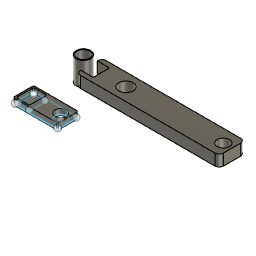
Chocolate Printer Parts v6 (Autodesk Fusion 360 design; units mm, degrees)
Autodesk Fusion 360 part; units mm, degrees
note: some values were not read from the file. Set by a fixed rule: which sketch regions a step uses.
sketch "Sketch1" plane through (0, 0, 0) normal (0, 0, 1) x (1, 0, 0)
  circle A0 centre (0, 0) radius 2.5
  circle A1 centre (0, 0) radius 3
  circle A2 centre (0, 0) radius 6
  circle A3 centre (0, 0) radius 7
  dimension "d1" = 5
  dimension "d2" = 0.5
  dimension "d5" = 12
  dimension "d6" = 1
  constraint coincident A0.centre A1.centre
  constraint concentric A0 A2
  measures "d1" diameter of A0
  measures "d5" diameter of A2
extrude "Extrude1" add sketch "Sketch1" along normal blind 10 contours A3 makes body 1
extrude "Extrude2" add sketch "Sketch1" against normal blind 5 contours A2 | A3 bodies 1
sketch "Sketch2" plane through (0, 0, 0) normal (0, 0, 1) x (1, 0, 0)
  line L0 (17, 5) -> (148.5, 5)
  line L1 (152.5, 1) -> (152.5, -16)
  line L2 (148.5, -20) -> (17, -20)
  line L3 (13, -16) -> (13, 1)
  line L4 (13, 0.5) -> (24, 0.5)
  line L5 (25, -0.5) -> (25, -14.5)
  line L6 (24, -15.5) -> (13, -15.5)
  line L7 (13, -15.5) -> (13, 0.5)
  circle A0 centre (49, -7.5) radius 6.5
  circle A1 centre (49, -7.5) radius 7
  circle A2 centre (144, -7.5) radius 6
  arc A3 (17, 5) -> (13, 1) centre (17, 1) ccw
  arc A4 (13, -16) -> (17, -20) centre (17, -16) ccw
  arc A5 (148.5, -20) -> (152.5, -16) centre (148.5, -16) ccw
  arc A6 (152.5, 1) -> (148.5, 5) centre (148.5, 1) ccw
  arc A7 (25, -0.5) -> (24, 0.5) centre (24, -0.5) ccw
  arc A8 (24, -15.5) -> (25, -14.5) centre (24, -14.5) ccw
  point P0 (12.5, -1.5)
  dimension "d9" = 25
  dimension "d10" = 16
  dimension "d11" = 4.5
  dimension "d12" = 4.5
  dimension "d13" = 12
  dimension "d14" = 24
  dimension "d15" = 13
  dimension "d16" = 0.5
  dimension "d17" = 95
  dimension "d18" = 12.5
  dimension "d19" = 12.5
  dimension "d20" = 12.5
  dimension "d21" = 12.5
  dimension "d22" = 12
  dimension "d39" = 4
  dimension "d40" = 4
  dimension "d41" = 1
  dimension "d47" = 8.5
  constraint horizontal L0
  constraint vertical L1
  constraint horizontal L2
  constraint vertical L3
  constraint horizontal L4
  constraint vertical L5
  constraint horizontal L6
  constraint vertical L7
  constraint coincident L3 L4.start
  constraint tangent L0 A3
  constraint tangent L3 A3
  constraint tangent L2 A4
  constraint tangent L3 A4
  constraint tangent L1 A5
  constraint tangent L2 A5
  constraint equal A4 A5
  constraint tangent L0 A6
  constraint tangent L1 A6
  constraint equal A4 A6
  constraint tangent L4 A7
  constraint tangent L5 A7
  constraint tangent L5 A8
  constraint tangent L6 A8
  constraint equal A7 A8
  measures "d9" distance of L0 L2
  measures "d10" distance of L4 L6
  measures "d11" distance of L0 L4
  measures "d12" distance of L2 L6
  measures "d13" distance of L3 L5
  measures "d14" distance of L5 A0.centre
  measures "d15" diameter of A0
  measures "d17" distance of A0.centre A2.centre
  measures "d18" distance of L0 A0.centre
  measures "d19" distance of L2 A0.centre
  measures "d20" distance of L2 A2.centre
  measures "d21" distance of L0 A2.centre
  measures "d22" diameter of A2
  measures "d39" radius of A3
  measures "d40" radius of A4
  measures "d41" radius of A7
  measures "d47" distance of L1 A2.centre
extrude "Extrude3" add sketch "Sketch2" along normal blind 11 separate body contours L0 L1 L2 L3 L4 L5 L6 A3 A4 A5 A6 A7 A8 makes body 2
sketch "Sketch3" plane through (0, 0, 0) normal (0, 0, 1) x (1, 0, 0)
  line L0 (-2.1132, -45.5462) -> (39.3868, -45.5462)
  line L1 (40.3868, -46.5462) -> (40.3868, -64.5462)
  line L2 (39.3868, -65.5462) -> (-2.1132, -65.5462)
  line L3 (-3.1132, -64.5462) -> (-3.1132, -46.5462)
  line L4 (-0.6132, -47.0462) -> (10.3868, -47.0462)
  line L5 (11.3868, -48.0462) -> (11.3868, -63.0462)
  line L6 (10.3868, -64.0462) -> (-0.6132, -64.0462)
  line L7 (-1.6132, -63.0462) -> (-1.6132, -48.0462)
  circle A0 centre (33.3868, -55.5462) radius 5.5
  arc A1 (-0.6132, -47.0462) -> (-1.6132, -48.0462) centre (-0.6132, -48.0462) ccw
  arc A2 (11.3868, -48.0462) -> (10.3868, -47.0462) centre (10.3868, -48.0462) ccw
  arc A3 (10.3868, -64.0462) -> (11.3868, -63.0462) centre (10.3868, -63.0462) ccw
  arc A4 (-1.6132, -63.0462) -> (-0.6132, -64.0462) centre (-0.6132, -63.0462) ccw
  arc A5 (-2.1132, -45.5462) -> (-3.1132, -46.5462) centre (-2.1132, -46.5462) ccw
  arc A6 (-3.1132, -64.5462) -> (-2.1132, -65.5462) centre (-2.1132, -64.5462) ccw
  arc A7 (39.3868, -65.5462) -> (40.3868, -64.5462) centre (39.3868, -64.5462) ccw
  arc A8 (40.3868, -46.5462) -> (39.3868, -45.5462) centre (39.3868, -46.5462) ccw
  dimension "d25" = 20
  dimension "d26" = 17
  dimension "d27" = 1.5
  dimension "d28" = 1.5
  dimension "d29" = 1.5
  dimension "d30" = 22
  dimension "d31" = 10
  dimension "d32" = 10
  dimension "d33" = 7
  dimension "d34" = 11
  dimension "d42" = 13
  dimension "d43" = 1
  dimension "d44" = 1
  constraint horizontal L0
  constraint vertical L1
  constraint horizontal L2
  constraint vertical L3
  constraint horizontal L4
  constraint vertical L5
  constraint horizontal L6
  constraint vertical L7
  constraint tangent L4 A1
  constraint tangent L7 A1
  constraint tangent L4 A2
  constraint tangent L5 A2
  constraint equal A1 A2
  constraint tangent L5 A3
  constraint tangent L6 A3
  constraint equal A1 A3
  constraint tangent L6 A4
  constraint tangent L7 A4
  constraint equal A1 A4
  constraint tangent L0 A5
  constraint tangent L3 A5
  constraint tangent L2 A6
  constraint tangent L3 A6
  constraint equal A5 A6
  constraint tangent L2 A7
  constraint tangent L1 A7
  constraint equal A5 A7
  constraint tangent L0 A8
  constraint tangent L1 A8
  constraint equal A5 A8
  measures "d25" distance of L0 L2
  measures "d26" distance of L4 L6
  measures "d27" distance of L0 L4
  measures "d28" distance of L3 L7
  measures "d29" distance of L2 L6
  measures "d30" distance of L5 A0.centre
  measures "d31" distance of L0 A0.centre
  measures "d32" distance of L2 A0.centre
  measures "d33" distance of L1 A0.centre
  measures "d34" diameter of A0
  measures "d42" distance of L5 L7
  measures "d43" radius of A1
  measures "d44" radius of A5
extrude "Extrude4" add sketch "Sketch3" along normal blind 5 separate body makes body 3
extrude "Extrude5" add sketch "Sketch3" against normal blind 1 contours L0 L1 L2 L3 A5 A6 A7 A8 | L4 L5 L6 L7 A1 A2 A3 A4 | A0 bodies 3
extrude "Extrude6" cut 1 faces at (36.2412, -54.5134, 0) along direction (0, 0, -1) blind 1 on bodies 3 bodies 3
sketch "Sketch4" plane through (0, 0, -5) normal (0, 0, -1) x (1, 0, 0)
  circle A0 centre (0, 0) radius 3
  circle A1 centre (0, 0) radius 7
  circle A2 centre (0, 0) radius 4
  dimension "d48" = 8
  constraint coincident A0.centre A1.centre
  measures "d48" diameter of A2
extrude "Extrude7" add sketch "Sketch4" along normal blind 8 contours A1 bodies 1
